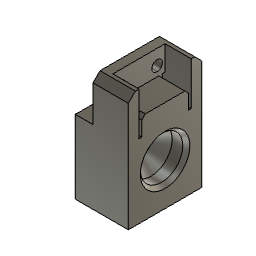
reset-tray v2 (Autodesk Fusion 360 design; units mm, degrees)
Autodesk Fusion 360 part; units mm, degrees
sketch "Sketch1" plane through (0, 0, 0) normal (0, 0, 1) x (1, 0, 0) in component "button-cage"
  line L0 (0, 0) -> (12, 0)
  line L1 (12, 0) -> (12, 10)
  line L2 (12, 10) -> (0, 10)
  line L3 (0, 10) -> (0, 0)
  dimension "d1" = 12
  dimension "d2" = 10
  constraint horizontal L0
  constraint vertical L1
  constraint horizontal L2
  constraint vertical L3
  constraint coincident L0.start L3.end
  measures "d1" distance of L0.start L0.end
  measures "d2" distance of L0.start L2.end
extrude "Extrude1" add sketch "Sketch1" along normal blind 5 makes body 1 in component "button-cage"
sketch "Sketch1 (2)" plane through (0, 0, 0) normal (-1, 0, 0) x (0, -1, 0) in component "button-cage"
  line L0 (-10, 0) -> (0, 0)
  line L1 (0, 0) -> (0, 5)
  line L2 (0, 5) -> (-10, 5)
  line L3 (-10, 5) -> (-10, 0)
  line L4 (-8.75, 1.25) -> (-1.25, 1.25)
  line L5 (-1.25, 1.25) -> (-1.25, 3.75)
  line L6 (-1.25, 3.75) -> (-8.75, 3.75)
  line L7 (-8.75, 3.75) -> (-8.75, 1.25)
  dimension "d5" = -1.25
extrude "Extrude2" cut sketch "Sketch1 (2)" against normal blind 10.5 contours L4 L5 L6 L7 bodies 1 in component "button-cage"
sketch "Sketch2" plane through (10.5, 0, 0) normal (-1, 0, 0) x (0, -1, 0) in component "button-cage"
  line L0 (-8.75, 3.75) -> (-8.75, 1.25)
  line L1 (-8.75, 1.25) -> (-1.25, 1.25)
  line L2 (-1.25, 1.25) -> (-1.25, 3.75)
  line L3 (-1.25, 3.75) -> (-8.75, 3.75)
  line L4 (-5, 3.75) -> (-5, 1.25) construction
  line L5 (-5, 2.5) -> (-3, 2.5) construction
  line L6 (-3, 2.5) -> (-3, 3.75) construction
  line L7 (-3, 3.75) -> (-7, 3.75) construction
  line L8 (-7, 3.75) -> (-7, 1.25) construction
  line L9 (-7, 1.25) -> (-3, 1.25) construction
  line L10 (-3, 1.25) -> (-3, 3.75) construction
  line L11 (-7, 1.25) -> (-3, 1.25)
  line L12 (-3, 1.25) -> (-3, 3.75)
  line L13 (-3, 3.75) -> (-7, 3.75)
  line L14 (-7, 3.75) -> (-7, 1.25)
  dimension "d8" = 2
  dimension "d9" = 4
  constraint midpoint L3 L4.start
  constraint midpoint L1 L4.end
  constraint midpoint L4 L5.start
  constraint perpendicular L4 L5
  constraint coincident L3 L6.end
  constraint perpendicular L3 L6
  constraint horizontal L7
  constraint vertical L8
  constraint horizontal L9
  constraint vertical L10
  constraint horizontal L11
  constraint vertical L12
  constraint horizontal L13
  constraint vertical L14
  measures "d8" distance of L5.start L5.end
  measures "d9" distance of L6.end L7.end
extrude "Extrude3" cut sketch "Sketch2" against normal up to surface (1.5 mm away) contours L1 L3 L11 L12 L13 L14 bodies 1 in component "button-cage"
fillet "Fillet1" radius 0.5 4 edges at (11.25, 3, 3.75) (11.25, 3, 1.25) (11.25, 7, 1.25) (11.25, 7, 3.75) on bodies 1 in component "button-cage"
chamfer "Chamfer1" distance 0.5 angle 45 8 edges at (12, 5, 3.75) (12, 6.8536, 3.6036) (12, 7, 2.5) (12, 6.8536, 1.3964) (12, 5, 1.25) (12, 3.1464, 1.3964) (12, 3, 2.5) (12, 3.1464, 3.6036) on bodies 1 in component "button-cage"
sketch "Sketch1 (3)" plane through (10.5, 0, 0) normal (-1, 0, 0) x (0, -1, 0) in component "button"
  line L0 (-7, 1.75) -> (-7, 3.25)
  arc A0 (-6.5, 3.75) -> (-7, 3.25) centre (-6.5, 3.25) ccw
  line L1 (-6.5, 3.75) -> (-8.75, 3.75)
  line L2 (-8.75, 3.75) -> (-8.75, 1.25)
  line L3 (-8.75, 1.25) -> (-6.5, 1.25)
  arc A1 (-7, 1.75) -> (-6.5, 1.25) centre (-6.5, 1.75) ccw
  line L4 (-3, 3.25) -> (-3, 1.75)
  arc A2 (-3.5, 1.25) -> (-3, 1.75) centre (-3.5, 1.75) ccw
  line L5 (-3.5, 1.25) -> (-1.25, 1.25)
  line L6 (-1.25, 1.25) -> (-1.25, 3.75)
  line L7 (-1.25, 3.75) -> (-3.5, 3.75)
  arc A3 (-3, 3.25) -> (-3.5, 3.75) centre (-3.5, 3.25) ccw
  line L8 (-8.75, 3.75) -> (-1.25, 3.75)
  line L9 (-1.25, 3.75) -> (-1.25, 1.25)
  line L10 (-1.25, 1.25) -> (-8.75, 1.25)
  line L11 (-8.75, 1.25) -> (-8.75, 3.75)
  constraint horizontal L8
  constraint vertical L9
  constraint horizontal L10
  constraint vertical L11
  constraint coincident L5.end L6.start
  constraint coincident L1.end L2.start
extrude "Extrude1'" add sketch "Sketch1 (3)" along normal blind 4 separate body makes body 2 in component "button"
sketch "Sketch2 (2)" plane through (10.5, 0, 0) normal (1, 0, 0) x (0, 1, 0) in component "button"
  line L0 (1.25, 1.25) -> (8.75, 1.25)
  line L1 (8.75, 1.25) -> (8.75, 3.75)
  line L2 (8.75, 3.75) -> (1.25, 3.75)
  line L3 (1.25, 3.75) -> (1.25, 1.25)
  arc A0 (3.5, 3.75) -> (3, 3.25) centre (3.5, 3.25) ccw
  line L4 (3, 1.75) -> (3, 3.25)
  arc A1 (3, 1.75) -> (3.5, 1.25) centre (3.5, 1.75) ccw
  line L5 (6.5, 1.25) -> (3.5, 1.25)
  arc A2 (6.5, 1.25) -> (7, 1.75) centre (6.5, 1.75) ccw
  line L6 (7, 3.25) -> (7, 1.75)
  arc A3 (7, 3.25) -> (6.5, 3.75) centre (6.5, 3.25) ccw
  line L7 (3.5, 3.75) -> (6.5, 3.75)
extrude "Extrude2'" add sketch "Sketch2 (2)" along normal blind 1.2 contours L0 L2 A0 L4 A1 L5 A2 L6 A3 L7 bodies 2 in component "button"
fillet "Fillet1'" radius 0.5 8 edges at (11.7, 3, 2.5) (11.7, 3.1464, 1.3964) (11.7, 5, 1.25) (11.7, 6.8536, 1.3964) (11.7, 7, 2.5) (11.7, 6.8536, 3.6036) (11.7, 5, 3.75) (11.7, 3.1464, 3.6036) on bodies 2 in component "button"
chamfer "Chamfer1'" distance 0.5 angle 45 4 edges at (8.5, 1.25, 3.75) (8.5, 1.25, 1.25) (8.5, 8.75, 3.75) (8.5, 8.75, 1.25) on bodies 2 in component "button"
sketch "Sketch1 (4)" plane through (0, 0, 0) normal (-1, 0, 0) x (0, -1, 0) in component "reset-button-retainer"
  line L0 (-1.25, 1.25) -> (-8.75, 1.25)
  line L1 (-8.75, 1.25) -> (-8.75, 3.75)
  line L2 (-8.75, 3.75) -> (-1.25, 3.75)
  line L3 (-1.25, 3.75) -> (-1.25, 1.25)
  line L4 (-10, 0) -> (0, 0)
  line L5 (0, 0) -> (0, 5)
  line L6 (0, 5) -> (-10, 5)
  line L7 (-10, 5) -> (-10, 0)
extrude "Extrude1''" add sketch "Sketch1 (4)" along normal blind 8 separate body makes body 3 in component "reset-button-retainer"
sketch "Sketch1 (5)" plane through (0, 0, 1.25) normal (0, 0, 1) x (-1, 0, 0) in component "reset-button"
  line L0 (0, -1.25) -> (0, -8.75)
  line L1 (0, -8.75) -> (8, -8.75)
  line L2 (8, -8.75) -> (8, -1.25)
  line L3 (8, -1.25) -> (0, -1.25)
  line L4 (19.5, -1) -> (12.1, -1)
  line L5 (12.1, -1) -> (12.1, -4.5)
  line L6 (12.1, -4.5) -> (19.5, -4.5)
  line L7 (19.5, -4.5) -> (19.5, -1)
  dimension "d24" = 7.4
  dimension "d25" = 3.5
  constraint horizontal L4
  constraint vertical L5
  constraint horizontal L6
  constraint vertical L7
  measures "d24" distance of L4.start L4.end
  measures "d25" distance of L4.start L6.end
extrude "Extrude1'''" add sketch "Sketch1 (5)" along normal blind 3.5 separate body contours L4 L5 L6 L7 makes body 4 in component "reset-button"
sketch "Sketch2 (3)" plane through (0, 0, 4.75) normal (0, 0, 1) x (-1, 0, 0) in component "reset-button"
  line L0 (19.5, -4.5) -> (19.5, -1)
  line L1 (19.5, -1) -> (12.1, -1)
  line L2 (12.1, -1) -> (12.1, -4.5)
  line L3 (12.1, -4.5) -> (19.5, -4.5)
  line L4 (19.5, -2.75) -> (12.1, -2.75) construction
  line L5 (15.8, -2.75) -> (15.8, -3.5) construction
  line L6 (15.8, -3.5) -> (17.3, -3.5) construction
  line L7 (17.3, -3.5) -> (14.3, -3.5)
  line L8 (14.3, -3.5) -> (14.3, -2)
  line L9 (14.3, -2) -> (17.3, -2)
  line L10 (17.3, -2) -> (17.3, -3.5)
  dimension "d28" = 0.75
  dimension "d29" = 1.5
  dimension "d30" = 3
  dimension "d31" = 1.5
  constraint midpoint L0 L4.start
  constraint midpoint L2 L4.end
  constraint midpoint L4 L5.start
  constraint perpendicular L4 L5
  constraint perpendicular L5 L6
  constraint horizontal L7
  constraint vertical L8
  constraint horizontal L9
  constraint vertical L10
  measures "d28" distance of L5.start L5.end
  measures "d29" distance of L5.end L6.end
  measures "d30" distance of L6.end L7.end
  measures "d31" distance of L6.end L9.end
extrude "Extrude2''" add sketch "Sketch2 (3)" along normal blind 1.25 contours L7 L8 L9 L10 bodies 4 in component "reset-button"
sketch "Sketch3" plane through (0, 1, 0) normal (0, -1, 0) x (1, 0, 0) in component "reset-button"
  line L0 (-19.5, 1.25) -> (-12.1, 1.25)
  line L1 (-12.1, 1.25) -> (-12.1, 4.75)
  line L2 (-12.1, 4.75) -> (-19.5, 4.75)
  line L3 (-19.5, 4.75) -> (-19.5, 1.25)
  line L4 (-12.1, 4.75) -> (-12.1, 2.75) construction
  line L5 (-12.1, 2.75) -> (-13.1, 2.75) construction
  line L6 (-19.5, 4.75) -> (-19.5, 2.75) construction
  line L7 (-19.5, 2.75) -> (-18.5, 2.75) construction
  line L8 (-18.5, 2.75) -> (-18.25, 2.75) construction
  line L9 (-18.25, 2.75) -> (-18.25, 2.5) construction
  line L10 (-18.25, 2.5) -> (-18.5, 2.5) construction
  line L11 (-18.5, 2.5) -> (-18.5, 2.75) construction
  line L12 (-13.1, 2.75) -> (-13.35, 2.75)
  line L13 (-13.35, 2.75) -> (-13.35, 2.5)
  line L14 (-13.35, 2.5) -> (-13.1, 2.5)
  line L15 (-13.1, 2.5) -> (-13.1, 2.75)
  line L16 (-18.5, 2.75) -> (-18.25, 2.75)
  line L17 (-18.25, 2.75) -> (-18.25, 2.5)
  line L18 (-18.25, 2.5) -> (-18.5, 2.5)
  line L19 (-18.5, 2.5) -> (-18.5, 2.75)
  dimension "d34" = 2
  dimension "d35" = 1
  dimension "d36" = 2
  dimension "d37" = 1
  dimension "d38" = 0.25
  dimension "d39" = 0.25
  dimension "d40" = 0.25
  dimension "d41" = 0.25
  constraint coincident L1.end L2.start
  constraint perpendicular L2 L4
  constraint perpendicular L1 L5
  constraint coincident L2.end L3.start
  constraint perpendicular L2 L6
  constraint perpendicular L3 L7
  constraint horizontal L8
  constraint vertical L9
  constraint horizontal L10
  constraint vertical L11
  constraint horizontal L12
  constraint vertical L13
  constraint horizontal L14
  constraint vertical L15
  constraint horizontal L16
  constraint vertical L17
  constraint horizontal L18
  constraint vertical L19
  measures "d34" distance of L1.end L4.end
  measures "d35" distance of L4.end L5.end
  measures "d36" distance of L2.end L6.end
  measures "d37" distance of L6.end L7.end
  measures "d38" distance of L7.end L8.end
  measures "d39" distance of L7.end L10.end
  measures "d40" distance of L5.end L12.end
  measures "d41" distance of L5.end L14.end
extrude "Extrude3'" add sketch "Sketch3" along normal blind 3.5 contours L12 L13 L14 L15 | L16 L17 L18 L19 bodies 4 in component "reset-button"
sketch "Sketch4" plane through (0, 0, 1.25) normal (0, 0, -1) x (1, 0, 0) in component "reset-button"
  line L0 (-19.5, -1) -> (-19.5, -4.5)
  line L1 (-19.5, -4.5) -> (-12.1, -4.5)
  line L2 (-12.1, -4.5) -> (-12.1, -1)
  line L3 (-12.1, -1) -> (-19.5, -1)
  line L4 (-19.5, -4.5) -> (-19.2, -4.5)
  line L5 (-19.2, -4.5) -> (-19.2, -1)
  line L6 (-12.1, -4.5) -> (-12.4, -4.5)
  line L7 (-12.4, -4.5) -> (-12.4, -1)
  dimension "d44" = 0.3
  dimension "d45" = 0.3
  constraint coincident L0.end L1.start
  constraint perpendicular L0 L4
  constraint coincident L3 L5.end
  constraint perpendicular L3 L5
  constraint coincident L1.end L2.start
  constraint perpendicular L2 L6
  constraint coincident L3 L7.end
  constraint perpendicular L3 L7
  measures "d44" distance of L0.end L4.end
  measures "d45" distance of L1.end L6.end
extrude "Extrude4" add sketch "Sketch4" along normal blind 2.5 separate body contours L0 L1 L3 L4 L5 | L1 L2 L3 L6 L7 makes body 5 at (-19.2, 3.3333, 0.4167) makes body 6 at (-12.1, 3.3333, 0.4167) in component "reset-button"
sketch "Sketch5" plane through (0, 1, 0) normal (0, -1, 0) x (1, 0, 0) in component "reset-button"
  line L0 (-19.2, 1.25) -> (-19.5, 1.25)
  line L1 (-19.5, 1.25) -> (-19.5, -1.25)
  line L2 (-19.5, -1.25) -> (-19.2, -1.25)
  line L3 (-19.2, -1.25) -> (-19.2, 1.25)
  line L4 (-12.1, 1.25) -> (-12.4, 1.25)
  line L5 (-12.4, 1.25) -> (-12.4, -1.25)
  line L6 (-12.4, -1.25) -> (-12.1, -1.25)
  line L7 (-12.1, -1.25) -> (-12.1, 1.25)
  line L8 (-19.5, -1.25) -> (-19.5, -1.15) construction
  line L9 (-19.5, -1.15) -> (-12.1, -1.15) construction
  line L10 (-19.5, -1.25) -> (-19.5, 0.35) construction
  line L11 (-19.5, 0.35) -> (-12.1, 0.35) construction
  line L12 (-12.1, 0.35) -> (-12.4, 0.35) construction
  line L13 (-19.2, 0.35) -> (-19.5, 0.35) construction
  line L14 (-19.5, -1.15) -> (-19.2, -1.15) construction
  line L15 (-12.4, -1.15) -> (-12.1, -1.15) construction
  line L16 (-19.5, 0.35) -> (-19.2, 0.35)
  line L17 (-19.2, 0.35) -> (-19.2, -1.25)
  line L18 (-19.2, -1.25) -> (-19.5, -1.25)
  line L19 (-19.5, -1.25) -> (-19.5, 0.35)
  line L20 (-19.5, 0.35) -> (-19.2, 0.35)
  line L21 (-19.2, 0.35) -> (-19.2, -1.15)
  line L22 (-19.2, -1.15) -> (-19.5, -1.15)
  line L23 (-19.5, -1.15) -> (-19.5, 0.35)
  line L24 (-12.4, 0.35) -> (-12.1, 0.35)
  line L25 (-12.1, 0.35) -> (-12.1, -1.15)
  line L26 (-12.1, -1.15) -> (-12.4, -1.15)
  line L27 (-12.4, -1.15) -> (-12.4, 0.35)
  line L28 (-12.4, 0.35) -> (-12.1, 0.35)
  line L29 (-12.1, 0.35) -> (-12.1, -1.25)
  line L30 (-12.1, -1.25) -> (-12.4, -1.25)
  line L31 (-12.4, -1.25) -> (-12.4, 0.35)
  dimension "d48" = 0.1
  dimension "d49" = 1.6
  constraint coincident L1.end L2.start
  constraint perpendicular L2 L8
  constraint coincident L7 L9.end
  constraint perpendicular L7 L9
  constraint perpendicular L2 L10
  constraint coincident L7 L11.end
  constraint perpendicular L7 L11
  constraint coincident L11 L12.end
  constraint coincident L5 L12.end
  constraint coincident L3 L13.start
  constraint coincident L11 L13.start
  constraint coincident L9 L14.end
  constraint coincident L3 L14.end
  constraint coincident L5 L15.start
  constraint coincident L9 L15.start
  constraint horizontal L16
  constraint vertical L17
  constraint horizontal L18
  constraint vertical L19
  constraint coincident L2.end L3.start
  constraint horizontal L20
  constraint vertical L21
  constraint horizontal L22
  constraint vertical L23
  constraint horizontal L24
  constraint vertical L25
  constraint horizontal L26
  constraint vertical L27
  constraint horizontal L28
  constraint vertical L29
  constraint horizontal L30
  constraint vertical L31
  constraint coincident L6.end L7.start
  measures "d48" distance of L1.end L8.end
  measures "d49" distance of L1.end L10.end
extrude "Extrude5" add sketch "Sketch5" along normal blind 0.2 contours L1 L2 L3 L17 L18 L19 L22 | L5 L6 L7 L26 L29 L30 L31 bodies 5 6 in component "reset-button"
extrude "Extrude6" add sketch "Sketch5" along normal blind 4.5 contours L1 L3 L16 L17 L19 L20 L21 L22 L23 | L5 L7 L24 L25 L26 L27 L28 L29 L31 bodies 5 6 in component "reset-button"
extrude "Extrude7" cut 2 faces at (-12.3, -0.5, 0.35) (-19.4, -0.5, 0.35) along direction (0, 0, -1) blind 0.5 on bodies 5 6 bodies 5 6 in component "reset-button"
sketch "Sketch6" plane through (0, 0.2327, 0) normal (0, -1, 0) x (1, 0, 0) in component "reset-button"
  line L0 (-10.7204, 13.0031) -> (-20.7204, 13.0031)
  line L1 (-20.7204, 13.0031) -> (-20.7204, 5.0031)
  line L2 (-20.7204, 5.0031) -> (-10.7204, 5.0031)
  line L3 (-10.7204, 5.0031) -> (-10.7204, 13.0031)
  line L4 (-11.9704, 13.0031) -> (-19.4704, 13.0031)
  line L5 (-19.4704, 13.0031) -> (-19.4704, 5.0031)
  line L6 (-19.4704, 5.0031) -> (-11.9704, 5.0031)
  line L7 (-11.9704, 5.0031) -> (-11.9704, 13.0031)
extrude "Extrude2'''" cut 1 faces at (-2.6667, 6.25, 3.75) along direction (0, 0, 1) blind 1.5 on bodies 3 bodies 3 in component "reset-button-retainer"
extrude "Extrude3''" add 1 faces at (-2.6667, 1.25, 3.75) along direction (0, 1, 0) blind 0.05 on bodies 3 bodies 3 in component "reset-button-retainer"
extrude "Extrude4'" add 1 faces at (-2.6667, 8.75, 2.5) along direction (0, -1, 0) blind 0.05 on bodies 3 bodies 3 in component "reset-button-retainer"
sketch "Sketch2 (4)" plane through (0, 0, 1.25) normal (0, 0, 1) x (-1, 0, 0) in component "reset-button-retainer"
  line L0 (0, -8.7) -> (8, -8.7)
  line L1 (8, -8.7) -> (8, -1.3)
  line L2 (8, -1.3) -> (0, -1.3)
  line L3 (0, -1.3) -> (0, -8.7)
  line L4 (4.9, -8.7) -> (4.9, -8.4)
  line L5 (4.9, -8.4) -> (5.9, -8.4)
  line L6 (5.9, -8.4) -> (5.9, -8.7)
  line L7 (5.9, -8.7) -> (4.9, -8.7)
  line L8 (4.9, -1.6) -> (4.9, -1.3)
  line L9 (4.9, -1.3) -> (5.9, -1.3)
  line L10 (5.9, -1.3) -> (5.9, -1.6)
  line L11 (5.9, -1.6) -> (4.9, -1.6)
extrude "Extrude5'" cut sketch "Sketch2 (4)" against normal blind 1.6 contours L0 L4 L5 L6 L7 | L2 L8 L9 L10 L11 bodies 3 in component "reset-button-retainer"
extrude "Extrude6'" cut 2 faces at (-4.9, 8.6, 0.8333) (-4.9, 1.5, 0.8333) along direction (1, 0, 0) blind 0.5 on bodies 3 bodies 3 in component "reset-button-retainer"
extrude "Extrude7'" cut 2 faces at (-5.9, 1.4, 0.8333) (-5.9, 8.5, 0.8333) along direction (-1, 0, 0) blind 0.5 on bodies 3 bodies 3 in component "reset-button-retainer"
chamfer "Chamfer1''" distance 1 angle 45 2 edges at (-4, 10, 5) (-4, 0, 5) on bodies 3 in component "reset-button-retainer"
sketch "Sketch3 (2)" plane through (0, 0, 0) normal (0, 0, -1) x (1, 0, 0) in component "reset-button-retainer"
  line L0 (-6.4, -1.3) -> (-4.4, -1.3)
  line L1 (-4.4, -1.3) -> (-4.4, -1.6)
  line L2 (-4.4, -1.6) -> (-6.4, -1.6)
  line L3 (-6.4, -1.6) -> (-6.4, -1.3)
  line L4 (-6.4, -8.4) -> (-4.4, -8.4)
  line L5 (-4.4, -8.4) -> (-4.4, -8.7)
  line L6 (-4.4, -8.7) -> (-6.4, -8.7)
  line L7 (-6.4, -8.7) -> (-6.4, -8.4)
  line L8 (0, -10) -> (0, 0)
  line L9 (0, 0) -> (-8, 0)
  line L10 (-8, 0) -> (-8, -10)
  line L11 (-8, -10) -> (0, -10)
  line L12 (-2.25, -7.7) -> (-2, -7.7)
  line L13 (-2, -7.7) -> (-2, -7.45)
  line L14 (-2, -7.45) -> (-2.25, -7.45)
  line L15 (-2.25, -7.45) -> (-2.25, -7.7)
  line L16 (-2.25, -2.3) -> (-2.25, -2.55)
  line L17 (-2.25, -2.55) -> (-2, -2.55)
  line L18 (-2, -2.55) -> (-2, -2.3)
  line L19 (-2, -2.3) -> (-2.25, -2.3)
  circle A0 centre (-2.125, -7.575) radius 0.5
  circle A1 centre (-2.125, -2.425) radius 0.5
  dimension "d69" = 1
  dimension "d70" = 1
  measures "d69" diameter of A0
  measures "d70" diameter of A1
extrude "Extrude8" cut sketch "Sketch3 (2)" against normal blind 1.5 contours L12 L13 L14 L15 | L16 L17 L18 L19 | A0 | A1 bodies 3 in component "reset-button-retainer"
sketch "Sketch1 (6)" plane through (0, 0, 0) normal (0, 0, 1) x (1, 0, 0) in component "v2"
sketch "Sketch1 (7)" plane through (0, 0, 0.9173) normal (0, 0, -1) x (1, 0, 0) in component "bracket"
  line L0 (-3.1265, -8.7) -> (0.3735, -8.7)
  line L1 (0.3735, -8.7) -> (0.3735, -1.3)
  line L2 (0.3735, -1.3) -> (-3.1265, -1.3)
  line L3 (-3.1265, -1.3) -> (-3.1265, -8.7)
extrude "Extrude1''''" add sketch "Sketch1 (7)" along normal blind 15 separate body makes body 7 in component "bracket"
extrude "Extrude2''''" add 1 faces at (-3.1265, 6.2333, -9.0827) along direction (-1, 0, 0) blind 4 on bodies 7 bodies 7 in component "bracket"
extrude "Extrude3'''" add 1 faces at (-2.1265, 1.3, -9.0827) along direction (0, -1, 0) blind 1.5 on bodies 7 bodies 7 in component "bracket"
extrude "Extrude4''" add 1 faces at (-2.1265, 8.7, -9.0827) along direction (0, 1, 0) blind 1.5 on bodies 7 bodies 7 in component "bracket"
extrude "Extrude5''" add 1 faces at (-2.1265, 3.2667, 0.9173) along direction (0, 0, 1) blind 3.5 on bodies 7 bodies 7 in component "bracket"
sketch "Sketch2 (5)" plane through (0.3735, 0, 0) normal (1, 0, 0) x (0, 1, 0) in component "bracket"
  line L0 (-0.2, 4.4173) -> (-0.2, -14.0827)
  line L1 (-0.2, -14.0827) -> (10.2, -14.0827)
  line L2 (10.2, -14.0827) -> (10.2, 4.4173)
  line L3 (10.2, 4.4173) -> (-0.2, 4.4173)
  line L4 (1.3, 0.9173) -> (8.7, 0.9173)
  line L5 (8.7, 0.9173) -> (8.7, 4.4173)
  line L6 (8.7, 4.4173) -> (1.3, 4.4173)
  line L7 (1.3, 4.4173) -> (1.3, 0.9173)
extrude "Extrude6''" cut sketch "Sketch2 (5)" against normal blind 3.7 contours L3 L4 L5 L6 L7 bodies 7 in component "bracket"
sketch "Sketch3 (3)" plane through (0.3735, 0, 0) normal (1, 0, 0) x (0, 1, 0) in component "bracket"
  line L0 (1.3, 0.9173) -> (1.3, 4.4173)
  line L1 (1.3, 4.4173) -> (-0.2, 4.4173)
  line L2 (-0.2, 4.4173) -> (-0.2, -14.0827)
  line L3 (-0.2, -14.0827) -> (10.2, -14.0827)
  line L4 (10.2, -14.0827) -> (10.2, 4.4173)
  line L5 (10.2, 4.4173) -> (8.7, 4.4173)
  line L6 (8.7, 4.4173) -> (8.7, 0.9173)
  line L7 (8.7, 0.9173) -> (1.3, 0.9173)
  line L8 (1.6, 0.9173) -> (1.3, 0.9173)
  line L9 (1.3, 0.9173) -> (1.3, -1.5827)
  line L10 (1.3, -1.5827) -> (1.6, -1.5827)
  line L11 (1.6, -1.5827) -> (1.6, 0.9173)
  line L12 (8.7, 0.9173) -> (8.4, 0.9173)
  line L13 (8.4, 0.9173) -> (8.4, -1.5827)
  line L14 (8.4, -1.5827) -> (8.7, -1.5827)
  line L15 (8.7, -1.5827) -> (8.7, 0.9173)
extrude "Extrude7''" cut sketch "Sketch3 (3)" against normal blind 8 contours L7 L8 L9 L10 L11 | L7 L12 L13 L14 L15 bodies 7 in component "bracket"
extrude "Extrude8'" cut 1 faces at (-3.3599, 1.6, -0.7493) along direction (0, 1, 0) blind 0.1 on bodies 7 bodies 7 in component "bracket"
extrude "Extrude9" cut 1 faces at (-3.3599, 8.4, -0.7493) along direction (0, -1, 0) blind 0.1 on bodies 7 bodies 7 in component "bracket"
extrude "Extrude10" cut 2 faces at (-2.1265, 1.4333, -1.5827) (-4.6265, 8.4333, -1.5827) along direction (0, 0, -1) blind 0.1 on bodies 7 bodies 7 in component "bracket"
sketch "Sketch4 (2)" plane through (-7.1265, 0, 0) normal (-1, 0, 0) x (0, -1, 0) in component "bracket"
  line L0 (-1.7, -1.6827) -> (-1.7, 0.9173)
  line L1 (-1.7, 0.9173) -> (-1.3, 0.9173)
  line L2 (-1.3, 0.9173) -> (-1.3, -1.6827)
  line L3 (-1.3, -1.6827) -> (-1.7, -1.6827)
  line L4 (-8.7, -1.6827) -> (-8.7, 0.9173)
  line L5 (-8.7, 0.9173) -> (-8.3, 0.9173)
  line L6 (-8.3, 0.9173) -> (-8.3, -1.6827)
  line L7 (-8.3, -1.6827) -> (-8.7, -1.6827)
  line L8 (-10.2, 4.4173) -> (-10.2, -14.0827)
  line L9 (-10.2, -14.0827) -> (0.2, -14.0827)
  line L10 (0.2, -14.0827) -> (0.2, 4.4173)
  line L11 (0.2, 4.4173) -> (-10.2, 4.4173)
  line L12 (-2.3, 2.1673) -> (-2.55, 2.1673)
  line L13 (-2.55, 2.1673) -> (-2.55, 2.4173)
  line L14 (-2.55, 2.4173) -> (-2.3, 2.4173)
  line L15 (-2.3, 2.4173) -> (-2.3, 2.1673)
  line L16 (-7.7, 2.1673) -> (-7.7, 2.4173)
  line L17 (-7.7, 2.4173) -> (-7.45, 2.4173)
  line L18 (-7.45, 2.4173) -> (-7.45, 2.1673)
  line L19 (-7.45, 2.1673) -> (-7.7, 2.1673)
  line L20 (-8.7, 0.9173) -> (-1.3, 0.9173)
  line L21 (-1.3, 0.9173) -> (-1.3, 4.4173)
  line L22 (-1.3, 4.4173) -> (-8.7, 4.4173)
  line L23 (-8.7, 4.4173) -> (-8.7, 0.9173)
  line L24 (-7.7, 2.1673) -> (-7.45, 2.4173) construction
  line L25 (-2.55, 2.1673) -> (-2.3, 2.4173) construction
  circle A0 centre (-7.575, 2.2923) radius 0.75 construction
  circle A1 centre (-7.575, 2.2923) radius 0.75
  circle A2 centre (-2.425, 2.2923) radius 0.75
  dimension "d93" = 1.5
  dimension "d94" = 1.5
  constraint coincident L16.start L19.end
  constraint coincident L17.end L18.start
  constraint coincident L12.end L13.start
  constraint coincident L14.end L15.start
  constraint midpoint L24 A0.centre
  constraint concentric A0 A1
  constraint midpoint L25 A2.centre
  measures "d93" diameter of A0
  measures "d94" diameter of A2
extrude "Extrude11" cut sketch "Sketch4 (2)" against normal blind 5 contours L12 L13 L14 L15 | L16 L17 L18 L19 | A1 | A2 bodies 7 in component "bracket"
extrude "Extrude12" cut sketch "Sketch4 (2)" against normal blind 2.5 contours L1 L5 L11 L20 L21 L22 L23 bodies 7 in component "bracket"
chamfer "Chamfer1'''" distance 1 angle 45 2 edges at (-3.3765, -0.2, 4.4173) (-3.3765, 10.2, 4.4173) on bodies 7 in component "bracket"
sketch "Sketch5 (2)" plane through (-7.1265, 0, 0) normal (-1, 0, 0) x (0, -1, 0) in component "bracket"
  line L0 (-9.2, 4.4173) -> (-10.2, 3.4173)
  line L1 (-10.2, 3.4173) -> (-10.2, -14.0827)
  line L2 (-10.2, -14.0827) -> (0.2, -14.0827)
  line L3 (0.2, -14.0827) -> (0.2, 3.4173)
  line L4 (0.2, 3.4173) -> (-0.8, 4.4173)
  line L5 (-0.8, 4.4173) -> (-1.3, 4.4173)
  line L6 (-1.3, 4.4173) -> (-1.3, -1.6827)
  line L7 (-1.3, -1.6827) -> (-1.7, -1.6827)
  line L8 (-1.7, -1.6827) -> (-1.7, 0.9173)
  line L9 (-1.7, 0.9173) -> (-8.3, 0.9173)
  line L10 (-8.3, 0.9173) -> (-8.3, -1.6827)
  line L11 (-8.3, -1.6827) -> (-8.7, -1.6827)
  line L12 (-8.7, -1.6827) -> (-8.7, 4.4173)
  line L13 (-8.7, 4.4173) -> (-9.2, 4.4173)
  line L14 (-8.7, -1.6827) -> (0.2, -1.6827)
  line L15 (-8.7, -1.6827) -> (-10.2, -1.6827)
  constraint coincident L11.end L12.start
  constraint coincident L3 L14.end
  constraint perpendicular L3 L14
  constraint coincident L1 L15.end
  constraint perpendicular L1 L15
extrude "Extrude13" cut sketch "Sketch5 (2)" against normal blind 2.5 contours L0 L1 L12 L13 L15 | L8 L9 L10 L14 | L3 L4 L5 L6 L14 bodies 7 in component "bracket"
sketch "Sketch6 (2)" plane through (0.3735, 0, 0) normal (1, 0, 0) x (0, 1, 0) in component "bracket"
  line L0 (10.2, 3.4173) -> (9.2, 4.4173)
  line L1 (9.2, 4.4173) -> (8.7, 4.4173)
  line L2 (8.7, 4.4173) -> (8.7, -1.6827)
  line L3 (8.7, -1.6827) -> (8.3, -1.6827)
  line L4 (8.3, -1.6827) -> (8.3, 0.9173)
  line L5 (8.3, 0.9173) -> (1.7, 0.9173)
  line L6 (1.7, 0.9173) -> (1.7, -1.6827)
  line L7 (1.7, -1.6827) -> (1.3, -1.6827)
  line L8 (1.3, -1.6827) -> (1.3, 4.4173)
  line L9 (1.3, 4.4173) -> (0.8, 4.4173)
  line L10 (0.8, 4.4173) -> (-0.2, 3.4173)
  line L11 (-0.2, 3.4173) -> (-0.2, -14.0827)
  line L12 (-0.2, -14.0827) -> (10.2, -14.0827)
  line L13 (10.2, -14.0827) -> (10.2, 3.4173)
  line L14 (5, -14.0827) -> (5, -3.0827) construction
  line L15 (5, -14.0827) -> (5, -11.5827) construction
  circle A0 centre (5, -11.5827) radius 1.5
  line L16 (5, -11.5827) -> (5, -6.1127) construction
  circle A1 centre (5, -6.1127) radius 1.5 construction
  circle A2 centre (5, -6.1127) radius 1.5
  circle A3 centre (5, -6.1127) radius 3
  circle A4 centre (5, -11.5827) radius 3
  circle A5 centre (5, -11.5827) radius 1.975
  dimension "d102" = 11
  dimension "d103" = 2.5
  dimension "d104" = 3
  dimension "d105" = 5.47
  dimension "d106" = 3
  dimension "d107" = 6
  dimension "d108" = 6
  dimension "d116" = 3.95
  constraint midpoint L12 L14.start
  constraint perpendicular L12 L14
  constraint perpendicular L12 L15
  constraint coincident L15.end A0.centre
  constraint parallel L14 L16
  constraint coincident L16.end A1.centre
  constraint concentric A2 A3
  constraint concentric A0 A4
  constraint concentric A0 A5
  measures "d102" distance of L14.start L14.end
  measures "d103" distance of L14.start L15.end
  measures "d104" diameter of A0
  measures "d105" distance of L15.end L16.end
  measures "d106" diameter of A1
  measures "d107" diameter of A3
  measures "d108" diameter of A4
  measures "d116" diameter of A5
extrude "Extrude16" add sketch "Sketch6 (2)" against normal blind 10.5 contours A0 | A5 bodies 7 in component "bracket"
extrude "Extrude14" cut sketch "Sketch6 (2)" against normal blind 12.5 contours A2 bodies 7 in component "bracket"
extrude "Extrude15" cut sketch "Sketch6 (2)" against normal blind 2 contours A3 A4 | A3 A4 bodies 7 in component "bracket"
chamfer "Chamfer2" distance 1.5 angle 45 1 edges at (-1.6265, 3.6015, -6.6551) on bodies 7 in component "bracket"
chamfer "Chamfer3" distance 0.5 angle 45 1 edges at (0.3735, 2.203, -5.0278) on bodies 7 in component "bracket"
chamfer "Chamfer4" distance 0.5 angle 45 1 edges at (-7.1265, 3.6015, -6.6551) on bodies 7 in component "bracket"
chamfer "Chamfer5" distance 0.5 angle 45 1 edges at (-10.1265, 3.1587, -10.8685) on bodies 7 in component "bracket"
chamfer "Chamfer6" distance 2 angle 45 2 edges at (-3.3765, -0.2, -14.0827) (-3.3765, 10.2, -14.0827) on bodies 7 in component "bracket"
chamfer "Chamfer7" distance 2 angle 45 1 edges at (0.3735, 5, -14.0827) on bodies 7 in component "bracket"
chamfer "Chamfer8" distance 0.5 angle 45 2 edges at (-1.4765, 1.7, 0.9173) (-1.4765, 8.3, 0.9173) on bodies 7 in component "bracket"
component "button-cage" placed x (1, 0, 0) y (0, 1, 0) z (0, 0, 1) at (0, 0, 0)
component "button" placed x (1, 0, 0) y (0, 1, 0) z (0, 0, 1) at (0, 0, 0)
component "reset-button-retainer" placed x (1, 0, 0) y (0, 1, 0) z (0, 0, 1) at (0, 0, 0)
component "v2" placed x (1, 0, 0) y (0, 1, 0) z (0, 0, 1) at (0, 0, 0)
component "reset-button" placed x (0, -1, 0) y (1, 0, 0) z (0, 0, 1) at (-4.1265, -10.8, -0.3327) in component "v2"
component "bracket" placed x (1, 0, 0) y (0, 1, 0) z (0, 0, 1) at (0, 0, 0) in component "v2"
